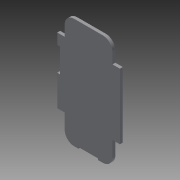
# Autodesk Inventor part: kryt_v1,1
Saved by Autodesk Inventor 2015 (Build 190159000, 159)
## iProperties
Created: 2016-01-01
Part Number: kryt_v1,1
Material: Generic
Document SubType Name: Modeling
Designer: Turboslimak
Density: 1 g/cm^3
Appearance: Default
Author: Turboslimak
Autodesk Inventor part; units mm, degrees
ref_plane "YZ Plane" through (0, 0, 0) normal (1, 0, 0) x (0, 1, 0)
ref_plane "XZ Plane" through (0, 0, 0) normal (0, 1, 0) x (-1, 0, 0)
ref_plane "XY Plane" through (0, 0, 0) normal (0, 0, 1) x (1, 0, 0)
sketch "Sketch1" plane through (0, 0, 0) normal (0, 1, 0) x (-1, 0, 0)
  line L0 (49.6, -114.5) -> (49.6, -63.5)
  line L1 (49.6, -63.5) -> (65, -63.5)
  line L2 (-65, -63.5) -> (-49.6, -63.5)
  line L3 (-49.6, -63.5) -> (-49.6, -114.5)
  line L4 (-65, 72.3) -> (-49.6, 72.3)
  line L5 (-65, -63.5) -> (-65, 72.3)
  line L6 (-49.6, 72.3) -> (-49.6, 114.5)
  line L7 (49.6, 114.5) -> (49.6, 72.3)
  line L8 (49.6, 72.3) -> (65, 72.3)
  line L9 (49.6, 114.5) -> (-49.6, 114.5)
  line L10 (49.6, -114.5) -> (21.2, -114.5)
  line L11 (21.2, -114.5) -> (21.2, -111.5)
  line L12 (-49.6, -114.5) -> (-19.6, -114.5)
  line L13 (-19.6, -114.5) -> (-19.6, -111.5)
  line L14 (-19.6, -111.5) -> (21.2, -111.5)
  line L15 (65, 72.3) -> (65, 50)
  line L16 (65, 50) -> (59, 50)
  line L17 (59, 50) -> (59, 0)
  line L18 (59, 0) -> (65, 0)
  line L19 (65, 0) -> (65, -63.5)
  point P0 (0, 0)
  dimension "d3" = 51
  dimension "d5" = 15.4
  dimension "d8" = 15.4
  dimension "d10" = 42.2
  dimension "d11" = 28.4
  dimension "d13" = 30
  dimension "d14" = 3
  dimension "d15" = 40.8
  dimension "d16" = 22.3
  dimension "d17" = 6
  dimension "d18" = 50
  constraints: 40 end point, 6 perpendicular, 2 horizontal, 1 vertical
  measures "d3" distance of L0.start L0.end
  measures "d5" distance of L2.start L2.end
  measures "d8" distance of L4.start L4.end
  measures "d10" distance of L7.start L7.end
  measures "d11" distance of L0.start L10.end
  measures "d13" distance of L3.end L12.end
  measures "d14" distance of L12.end L13.end
  measures "d15" distance of L13.end L11.end
  measures "d16" distance of L8.end L15.end
  measures "d17" distance of L15.end L16.end
  measures "d18" distance of L16.end L17.end
extrude "Extrusion1" add sketch "Sketch1" along normal blind 6
fillet "Fillet1" radius 20 4 edges at (49.6, 3, -114.5) (-49.6, 3, -114.5) (49.6, 3, 114.5) (-49.6, 3, 114.5)
body "Solid1"
